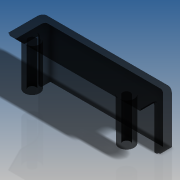
# Autodesk Inventor part: 11235-TransBlackIRLens
Saved by Autodesk Inventor 2016 SP2 (Build 200236200, 236)
## iProperties
Created: 2015-08-26
Part Number: 11235-TransBlackIRLens
Material: Polycarbonate
Document SubType Name: Modeling
Designer: D. Kohfeld
Density: 1.2 g/cm^3
Appearance: TransBlackIRLens
Mass: 1.48877 g
Surface Area: 22.7172 cm^2
Volume: 1.24064 cm^3
Author: D. Kohfeld
Autodesk Inventor part; units mm, degrees
ref_plane "YZ Plane" through (0, 0, 0) normal (1, 0, 0) x (0, 1, 0)
ref_plane "XZ Plane" through (0, 0, 0) normal (0, 1, 0) x (-1, 0, 0)
sketch "Sketch2" plane through (0, 0, 0) normal (1, 0, 0) x (0, 1, 0)
  line L0 (-10.8, -4.8) -> (1.2, -4.8)
  arc A0 (1.2, -4.8) -> (4.8, -1.2) centre (1.2, -1.2) ccw
  line L1 (4.8, -1.2) -> (4.8, 6.4)
  line L2 (4.8, 6.4) -> (4.4, 6.4)
  line L3 (4.4, 6.4) -> (1.2, 3.2)
  line L4 (1.2, 3.2) -> (1.2, 0)
  arc A1 (0, -1.2) -> (1.2, 0) centre (0, 0) ccw
  line L5 (0, -1.2) -> (-10.8, -1.2)
  line L6 (-10.8, -1.2) -> (-10.8, -4.8)
  line L7 (3.6, 5.6) -> (3.6, -1.2)
  arc A2 (1.2, -3.6) -> (3.6, -1.2) centre (1.2, -1.2) ccw
  line L8 (1.2, -3.6) -> (-10.8, -3.6)
  dimension "d0" = 3.6
  dimension "d1" = 1.2
  dimension "d2" = 45
  dimension "d3" = 1.2
  dimension "d4" = 3.6
  dimension "d5" = 15.6
  dimension "d6" = 0.4
  dimension "d7" = 3.6
  dimension "d9" = 11.2
  constraints: 18 end point, 6 point on circle, 6 tangent, 4 horizontal, 4 vertical, 3 centre point, 2 point on line, 1 coincident, 1 concentric
  measures "d0" distance between parallel lines of L1 L4
  measures "d1" distance between parallel lines of L1 L7
  measures "d2" angle of L3 L4
  measures "d3" radius of A1
  measures "d4" distance between parallel lines of L5 L0
  measures "d5" distance between parallel lines of L6 L1
  measures "d6" distance from line of L1 L2.end
  measures "d7" radius of A0
  measures "d9" distance from line of L0 L1.end
extrude "Extrusion1" add sketch "Sketch2" along normal mid plane 32
extrude "Extrusion2" cut sketch "Sketch2" along normal mid plane 29.6 contours L6 L5 A1 L4 L3 L7 A2 L8
ref_plane "Work Plane1" through (-14.8, -7.6, 5.6) normal (0, -1, 0) x (1, 0, 0)
sketch "Sketch3" plane through (-14.8, -7.6, 5.6) normal (0, -1, 0) x (1, 0, 0)
  line L0 (29.6, -9.2) -> (0, -9.2) projected
  circle A0 centre (2.4, -2) radius 2
  circle A1 centre (2.4, -2) radius 1
  circle A2 centre (27.2, -2) radius 1
  circle A3 centre (27.2, -2) radius 2
  line L1 (2.4, -2) -> (27.2, -2) construction
  point P0 (14.8, -5.6)
  point P1 (14.8, -2)
  dimension "d15" = 24.8
  dimension "d16" = 4
  dimension "d17" = 2
  dimension "d18" = 7.2
  constraints: 4 centre point, 2 coincident, 2 end point, 2 equal radius, 1 horizontal, 1 midpoint, 1 vertical alignment
  measures "d15" distance of L1.start L1.end
  measures "d16" diameter of A0
  measures "d17" diameter of A1
  measures "d18" distance between parallel lines of L0 L1
extrude "Extrusion3" add sketch "Sketch3" against normal up to next
sketch "Sketch4" plane through (16, 0, 0) normal (1, 0, 0) x (0, 0, -1)
  line L0 (-6.4, 4.8) -> (-6.4, 4.4) projected
  line L1 (-6.4, 4.4) -> (-3.2, 1.2) projected
  line L2 (-3.2, 1.2) -> (0, 1.2) projected
  arc A0 (1.2, 0) -> (0, 1.2) centre (0, 0) ccw projected
  line L3 (1.2, 0) -> (1.2, -10.8) projected
  line L4 (1.2, -10.8) -> (4.8, -10.8) projected
  line L5 (-6.4, 4.8) -> (-3.2, 1.6)
  line L6 (-3.2, 1.6) -> (0, 1.6)
  arc A1 (1.6, 0) -> (0, 1.6) centre (0, 0) ccw
  line L7 (1.6, 0) -> (1.6, -10.8)
  dimension "d21" = 0.4
  constraints: 6 end point, 2 point on circle, 2 tangent, 1 centre point, 1 concentric, 1 horizontal, 1 parallel, 1 point on line, 1 vertical
  measures "d21" distance between parallel lines of L3 L7
extrude "Extrusion4" cut sketch "Sketch4" against normal blind 0.4
mirror "Mirror1" about plane through (0, 0, 0) normal (1, 0, 0) of "Extrusion4"
fillet "Fillet1" radius 0.1 54 edges at (0, 4.4, 6.4) (10.4, -7.6, 3.6) (-14.4, -7.6, 3.6) (15.2, -10.8, -1.2) (14.8, 0.8485, -0.8485) (14.8, 1.2, 1.6) (14.8, -5.4, -1.2) (15.6, 0.8485, -0.8485) (15.6, 1.2, 1.6) (15.6, -5.4, -1.2) (16, 1.1314, -1.1314) (16, 1.6, 1.6) (16, -5.4, -1.6) (15.6, -10.8, -1.4) (15.8, -10.8, -1.6) (16, -10.8, -3.2) (0, -10.8, -4.8) (16, 3.7456, -3.7456) (16, 4.8, 2.6) (16, -4.8, -4.8) (16, 3.2, 4.8) (15.6, 2.8, 4.8) (15.6, 4.6, 6.4) (14.8, -10.8, -2.4) (0, -10.8, -3.6) (-14.8, -10.8, -2.4) (15.8, 1.6, 3.2) (15.2, 1.2, 3.2) (14.8, 2.4, 4.4) (13.6, 3.6, 5.6) (0, 3.6, 5.6) (-13.6, 3.6, 5.6) (-14.8, 2.4, 4.4) (-15.6, 2.8, 4.8) (-15.6, 4.6, 6.4) (-16, 3.7456, -3.7456) (-16, -4.8, -4.8) (-16, 4.8, 2.6) (-16, -10.8, -3.2) (-15.8, -10.8, -1.6) (-16, 1.1314, -1.1314) (-16, 1.6, 1.6) (-16, -5.4, -1.6) (-15.6, -10.8, -1.4) (-15.6, 0.8485, -0.8485) (-15.6, 1.2, 1.6) (-15.6, -5.4, -1.2) (-15.2, -10.8, -1.2) (-14.8, 0.8485, -0.8485) (-14.8, 1.2, 1.6) (-14.8, -5.4, -1.2) (-16, 3.2, 4.8) (-15.8, 1.6, 3.2) (-15.2, 1.2, 3.2)
equation "\"d4\" = d0"
equation "\"d10\" = 4 * lu"
equation "\"lu\" = 8"
body "Solid1"
